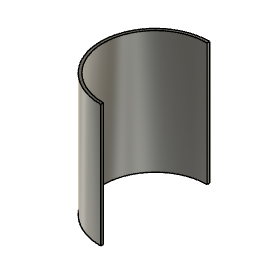
Vandana_SingleCylinderEngine v3 (Autodesk Fusion 360 archive; units mm, degrees)
design "8"
Autodesk Fusion 360 part; units mm, degrees
sketch "Sketch1" plane through (0, 0, 0) normal (0, 0, 1) x (1, 0, 0) in component "Component8"
  arc A0 (0, 55) -> (0, -55) centre (0, 0) ccw
  arc A1 (0, 57.73) -> (0, -57.73) centre (0, 0) ccw
  line L0 (0, 57.73) -> (0, 55)
  line L1 (0, -55) -> (0, -57.73)
  dimension "d1" = 55
  dimension "d2" = 57.73
  constraint coincident A0.centre A1.centre
  constraint vertical L0
  constraint parallel L0 L1
  measures "d1" radius of A0
  measures "d2" radius of A1
extrude "Extrude1" add sketch "Sketch1" along normal blind 130 in component "Component8"
component "Component8" placed x (1, 0, 0) y (0, 1, 0) z (0, 0, 1) at (0, 0, 0)

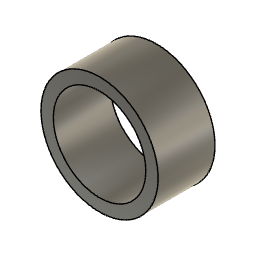
design "7"
Autodesk Fusion 360 part; units mm, degrees
sketch "Sketch1" plane through (0, 0, 0) normal (0, 1, 0) x (1, 0, 0) in component "Component7"
  circle A0 centre (0, 0) radius 30.885
  circle A1 centre (0, 0) radius 24.375
  dimension "d1" = 61.77
  dimension "d2" = 48.75
  constraint coincident A0.centre A1.centre
  constraint concentric A0 A1
  measures "d1" diameter of A0
  measures "d2" diameter of A1
extrude "Extrude1" add sketch "Sketch1" along normal blind 30 in component "Component7"
component "Component7" placed x (1, 0, 0) y (0, 1, 0) z (0, 0, 1) at (0, 0, 0)

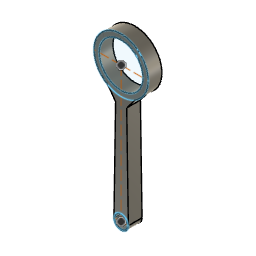
design "5"
Autodesk Fusion 360 part; units mm, degrees
sketch "Sketch1" plane through (0, 0, 0) normal (0, 1, 0) x (1, 0, 0) in component "Component5"
  circle A0 centre (0, -20) radius 31.975
  circle A1 centre (0, -20) radius 39.52
  line L0 (0, -20) -> (0, 177.87) construction
  circle A2 centre (0, 177.87) radius 9.5
  circle A3 centre (0, 177.87) radius 10.5
  line L1 (0, 177.87) -> (10.5, 177.87) construction
  line L2 (0, 177.87) -> (-10.5, 177.87) construction
  line L3 (0, -20) -> (39.52, -20) construction
  line L4 (0, -20) -> (-39.52, -20) construction
  dimension "d1" = 63.95
  dimension "d2" = 79.04
  dimension "d3" = 197.87
  dimension "d4" = 19
  dimension "d5" = 21
  constraint concentric A0 A1
  constraint coincident A0.centre A1.centre
  constraint vertical L0
  constraint coincident L0.end A2.centre
  constraint concentric A2 A3
  constraint coincident A3 L1.end
  constraint perpendicular L0 L1
  constraint coincident A3 L2.end
  constraint perpendicular L0 L2
  constraint coincident A1 L3.end
  constraint perpendicular L0 L3
  constraint coincident A1 L4.end
  constraint perpendicular L0 L4
  measures "d1" diameter of A0
  measures "d2" diameter of A1
  measures "d3" distance of A0.centre L0.end
  measures "d4" diameter of A2
  measures "d5" diameter of A3
sketch "Sketch2" plane through (0, 0, 0) normal (0, 1, 0) x (1, 0, 0) in component "Component5"
  line L0 (-10.5014, 177.87) -> (-8.1004, 29.9645)
  line L1 (-10.5014, 177.87) -> (137.425, 177.87) construction
  line L2 (10.5014, 177.87) -> (8.1008, 29.9845)
  line L3 (10.5014, 177.87) -> (158.3855, 177.87) construction
  line L4 (8.1008, 29.9845) -> (20.0649, 14.0475)
  line L5 (-8.1004, 29.9645) -> (-20.0795, 14.0388)
  circle A0 centre (0, 177.87) radius 10.5
  circle A1 centre (0, -20) radius 39.52
  dimension "d6" = 89.07
  dimension "d7" = 147.9055
  dimension "d8" = 90.93
  dimension "d9" = 147.905
  dimension "d10" = 19.9281
  dimension "d12" = 19.928
  constraint horizontal L1
  constraint horizontal L3
  constraint coincident L1 L2.start
  constraint tangent L2 A0
  constraint tangent L0 A0
  constraint coincident L4.end A1
  constraint coincident L5.end A1
  measures "d6" angle of L0 L1
  measures "d7" vertical distance of L0.start L0.end
  measures "d8" angle of L2 L3
  measures "d9" distance of L2.start L2.end
  measures "d10" distance of L2.end L4.end
  measures "d12" distance of L0.end L5.end
extrude "Extrude1" add sketch "Sketch2" along normal blind 20 contours L0 L2 L4 L5 A0 A1 | A0 | A1 in component "Component5"
extrude "Extrude2" cut sketch "Sketch1" along normal blind 20 contours A0 in component "Component5"
extrude "Extrude3" cut sketch "Sketch1" along normal blind 20 contours A2 in component "Component5"
component "Component5" placed x (1, 0, 0) y (0, 1, 0) z (0, 0, 1) at (0, 0, 0)
